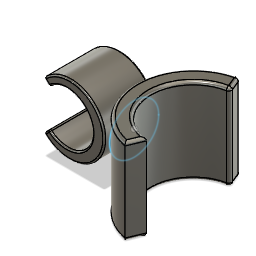
exposure_ligt_mount (Autodesk Fusion 360 design; units mm, degrees)
Autodesk Fusion 360 part; units mm, degrees
other "Base Mesh Feature1"
other "MeshRepair1"
sketch "Sketch1" plane through (0, 0, 0) normal (0, 0, 1) x (1, 0, 0)
  circle A0 centre (-18.3865, -6.1523) radius 17.1081
  circle A1 centre (-19.6932, -6.1528) radius 12.6163
  line L0 (-28.2753, 3.0949) -> (-30.8023, 5.6179)
  line L1 (-28.2753, -15.4004) -> (-30.8023, -17.9225)
  constraint coincident A1 L0.start
  constraint coincident A0 L0.end
  constraint coincident A1 L1.start
  constraint coincident A0 L1.end
extrude "Extrude1" add sketch "Sketch1" along normal blind 25 contours A0 A1 L0 L1 picked at (-3.5696, -9.2796) makes body 1
scale "Scale1" factor 0.7137 about (-30.8023, 5.6179, 0) bodies 1
fillet "Fillet1" radius 0.5 12 edges at (-28.9988, 3.8172, 8.9212) (-29.9005, 4.7176, 17.8425) (-30.8023, 5.6179, 8.9212) (-29.9005, 4.7176, 0) (-30.8023, -11.1829, 8.9212) (-28.9988, -9.3829, 8.9212) (-9.7311, -2.7825, 17.8425) (-29.9005, -10.2829, 17.8425) (-13.8695, -2.7828, 17.8425) (-13.8695, -2.7828, 0) (-9.7311, -2.7825, 0) (-29.9005, -10.2829, 0) on bodies 1
other "Modify1"
other "Modify2"
sketch "Sketch2" plane through (0, 0, 0) normal (0, 1, 0) x (1, 0, 0)
  circle A0 centre (14.8322, -8.7271) radius 20.4966
  circle A1 centre (14.6376, -8.7275) radius 14.8021
  line L0 (10.772, 11.3633) -> (12.9995, 5.9837)
  line L1 (12.9995, -23.4387) -> (10.772, -28.8175)
  constraint coincident A0 L0.start
  constraint coincident A1 L0.end
  constraint coincident A1 L1.start
  constraint coincident A0 L1.end
extrude "Extrude2" add sketch "Sketch2" along normal mid plane 30 separate body contours A0 A1 L0 L1 picked at (9.8576, 9.1742) makes body 2
move_body "Move1" bodies 1 to x (1, 0, 0) y (0, 1, 0) z (0, 0, 1) at (1.272, 3.0211, 0)
fillet "Fillet2" radius 1 10 edges at (-5.6644, 15, 8.7271) (-0.1645, 15, 8.7275) (10.772, 0, -11.3633) (12.9995, 0, -5.9837) (11.8857, 15, -8.6735) (11.8857, 15, 26.1281) (-5.6644, -15, 8.7271) (-0.1645, -15, 8.7275) (11.8857, -15, -8.6735) (11.8857, -15, 26.1281) on bodies 2
ref_plane "WorkPlane1" through (-6.8, 0, 0) normal (1, 0, 0) x (0, 1, 0)
sketch "Sketch3" plane through (-6.8, 0, 0) normal (1, 0, 0) x (0, 0, -1)
  circle A0 centre (-8, 0) radius 8.6023
move_body "Move2" bodies 1 to x (1, 0, 0) y (0, 1, 0) z (0, 0, 1) at (0, 0, -1)
